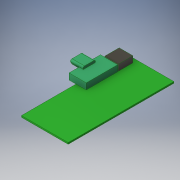
# Autodesk Inventor part: ControlBoard
Saved by Autodesk Inventor 2016 (Build 200138000, 138)
## iProperties
Created: 2016-08-11
Part Number: ControlBoard
Material: Generic
Document SubType Name: Modeling
Designer: jfixelle
Density: 1 g/cm^3
Appearance: Smooth - Dark Forest Green
Author: jfixelle
Autodesk Inventor part; units mm, degrees
ref_plane "YZ Plane" through (0, 0, 0) normal (1, 0, 0) x (0, 1, 0)
ref_plane "XZ Plane" through (0, 0, 0) normal (0, 1, 0) x (-1, 0, 0)
ref_plane "XY Plane" through (0, 0, 0) normal (0, 0, 1) x (1, 0, 0)
sketch "Sketch1" plane through (0, 0, 0) normal (0, 1, 0) x (-1, 0, 0)
  line L0 (24.13, 54.61) -> (-24.13, 54.61)
  line L1 (-24.13, 54.61) -> (-24.13, -54.61)
  line L2 (-24.13, -54.61) -> (24.13, -54.61)
  line L3 (24.13, -54.61) -> (24.13, 54.61)
  point P0 (0, 0)
  dimension "d0" = 109.22
  dimension "d1" = 48.26
  dimension "d4" = 24.13
  dimension "d5" = 54.61
  constraints: 8 end point, 2 parallel, 1 horizontal, 1 perpendicular
  measures "d0" distance of L2.end L0.start
  measures "d1" distance of L1.end L2.end
  measures "d4" distance from line of L1 point (0, 0)
  measures "d5" distance from line of L2 point (0, 0)
extrude "Extrusion1" add sketch "Sketch1" along normal blind 1.6
sketch "Sketch2" plane through (0, 1.6, 0) normal (0, 1, 0) x (1, 0, 0)
  line L0 (-13.716, 50.165) -> (-27.94, 50.165)
  line L1 (-27.94, 50.165) -> (-27.94, 35.179)
  line L2 (-27.94, 35.179) -> (-13.716, 35.179)
  line L3 (-13.716, 35.179) -> (-13.716, 50.165)
  line L4 (-24.13, 54.61) -> (-24.13, -54.61) projected
  line L5 (24.13, 54.61) -> (-24.13, 54.61) projected
  point P0 (0, 0)
  dimension "d6" = 14.224
  dimension "d7" = 14.986
  dimension "d8" = 3.81
  dimension "d9" = 4.445
  constraints: 8 end point, 2 parallel, 1 horizontal, 1 perpendicular
  measures "d6" distance of L1.end L2.end
  measures "d7" distance of L0.end L1.end
  measures "d8" distance between parallel lines of L4 L1
  measures "d9" distance between parallel lines of L5 L0
extrude "Extrusion2" add sketch "Sketch2" along normal blind 6.35
sketch "Sketch3" plane through (0, 1.6, 0) normal (0, 1, 0) x (1, 0, 0)
  line L0 (-31.369, 1.778) -> (-13.589, 1.778)
  line L1 (-13.589, 1.778) -> (-13.589, 34.29)
  line L2 (-13.589, 34.29) -> (-31.369, 34.29)
  line L3 (-31.369, 34.29) -> (-31.369, 1.778)
  line L4 (24.13, 54.61) -> (-24.13, 54.61) projected
  line L5 (-24.13, 35.179) -> (-24.13, -54.61) projected
  point P0 (0, 0)
  dimension "d12" = 32.512
  dimension "d13" = 17.78
  dimension "d14" = 20.32
  dimension "d15" = 7.239
  constraints: 8 end point, 2 parallel, 1 horizontal, 1 perpendicular
  measures "d12" distance of L2.end L0.start
  measures "d13" distance of L0.start L0.end
  measures "d14" distance between parallel lines of L4 L2
  measures "d15" distance between parallel lines of L5 L3
extrude "Extrusion3" add sketch "Sketch3" along normal blind 6.35
sketch "Sketch4" plane through (-31.369, 1.6, -34.29) normal (-1, 0, 0) x (0, 0, 1)
  line L0 (11.6254, 3.2104) -> (20.2625, 3.2104)
  line L1 (20.2625, 3.2104) -> (23.564, 8.9287)
  line L2 (23.564, 8.9287) -> (8.324, 8.9287)
  line L3 (8.324, 8.9287) -> (11.6254, 3.2104)
  point P0 (34.29, -1.6)
  dimension "d18" = 120
  dimension "d19" = 120
  dimension "d20" = 15.24
  constraints: 8 end point, 2 horizontal
  measures "d18" angle of L0 L3
  measures "d19" angle of L1 L0
  measures "d20" distance of L1.end L2.end
extrude "Extrusion4" add sketch "Sketch4" along normal blind 8.636 and the other way blind 4.318
fillet "Fillet1" radius 1.5875 4 edges at (-33.528, 10.5287, -25.966) (-33.528, 10.5287, -10.726) (-35.687, 4.8104, -22.6646) (-35.687, 4.8104, -14.0275)
body "Solid1"
